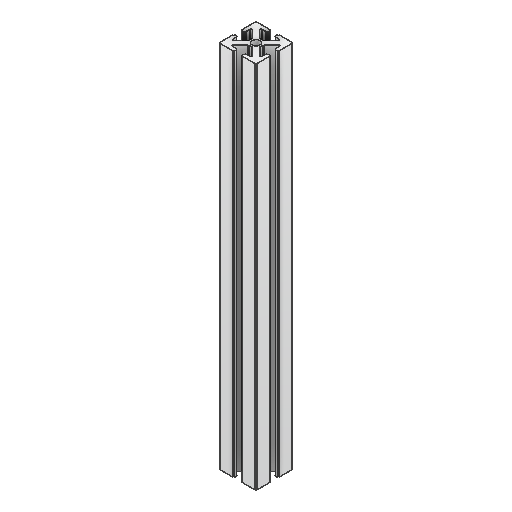
# Autodesk Inventor part: Strut_short
Saved by Autodesk Inventor 2025.2 (Build 292293000, 293)
## iProperties
Created: 2024-10-24
Part Number: Strut_short
Material: Generic
Document SubType Name: Modeling
Designer: rolan
Density: 1 g/cm^3
Appearance: Default
Author: rolan
Autodesk Inventor part; units mm, degrees
ref_plane "YZ Plane" through (0, 0, 0) normal (1, 0, 0) x (0, 1, 0)
ref_plane "XZ Plane" through (0, 0, 0) normal (0, 1, 0) x (-1, 0, 0)
ref_plane "XY Plane" through (0, 0, 0) normal (0, 0, 1) x (1, 0, 0)
sketch "Sketch1" plane through (0, 0, 0) normal (0, 1, 0) x (-1, 0, 0)
  line L0 (2.5, 10) -> (9.5, 10) construction
  line L1 (10, -2.5) -> (10, -9.5) construction
  line L2 (-2.5, -10) -> (-9.5, -10) construction
  line L3 (-10, 2.5) -> (-10, 10) construction
  line L4 (-10, 10) -> (10, -10) construction
  line L5 (10, 10) -> (-10, -10) construction
  circle A0 centre (0, 0) radius 2.15
  line L6 (10, 9.5) -> (10, 2.5)
  line L7 (9.5, 2) -> (8.5, 2)
  line L8 (8, 2.5) -> (8, 4.7929)
  line L9 (-0.7929, 3) -> (0.7929, 3)
  line L10 (3, 0.7929) -> (3, -0.7929)
  line L11 (0.7929, -3) -> (-0.7929, -3)
  line L12 (-3, -0.7929) -> (-3, 0.7929)
  line L13 (-3, 3) -> (3, -3) construction
  line L14 (3, 3) -> (-3, -3) construction
  line L15 (10, -10) -> (10, -2)
  line L16 (9.5, -2) -> (8.5, -2)
  line L17 (8, -2.5) -> (8, -4.7929)
  line L18 (7.1464, -5.1464) -> (3.1464, -1.1464)
  line L19 (7.1464, 5.1464) -> (3.1464, 1.1464)
  line L20 (8, 6) -> (13.6569, 6) construction
  line L21 (10, 10) -> (2, 10)
  line L22 (2, 9.5) -> (2, 8.5)
  line L23 (2.5, 8) -> (4.7929, 8)
  line L24 (5.1464, 7.1464) -> (1.1464, 3.1464)
  line L25 (-9.5, 10) -> (-2.5, 10)
  line L26 (-2, 9.5) -> (-2, 8.5)
  line L27 (-2.5, 8) -> (-4.7929, 8)
  line L28 (-5.1464, 7.1464) -> (-1.1464, 3.1464)
  line L29 (-10, 9.5) -> (-10, 2)
  line L30 (-9.5, 2) -> (-8.5, 2)
  line L31 (-8, 2.5) -> (-8, 4.7929)
  line L32 (-7.1464, 5.1464) -> (-3.1464, 1.1464)
  line L33 (-10, -9.5) -> (-10, -2.5)
  line L34 (-9.5, -2) -> (-8.5, -2)
  line L35 (-8, -2.5) -> (-8, -4.7929)
  line L36 (-7.1464, -5.1464) -> (-3.1464, -1.1464)
  line L37 (-8, -6) -> (-2.3431, -6) construction
  line L38 (-10, -10) -> (-2, -10)
  line L39 (-2, -9.5) -> (-2, -8.5)
  line L40 (-2.5, -8) -> (-4.7929, -8)
  line L41 (-5.1464, -7.1464) -> (-1.1464, -3.1464)
  line L42 (9.5, -10) -> (2.5, -10)
  line L43 (2, -9.5) -> (2, -8.5)
  line L44 (2.5, -8) -> (4.7929, -8)
  line L45 (5.1464, -7.1464) -> (1.1464, -3.1464)
  arc A1 (8, 2.5) -> (8.5, 2) centre (8.5, 2.5) ccw
  arc A2 (9.5, 2) -> (10, 2.5) centre (9.5, 2.5) ccw
  arc A3 (10, -2.5) -> (9.5, -2) centre (9.5, -2.5) ccw
  arc A4 (8.5, -2) -> (8, -2.5) centre (8.5, -2.5) ccw
  arc A5 (7.1464, -5.1464) -> (8, -4.7929) centre (7.5, -4.7929) ccw
  arc A6 (3, -0.7929) -> (3.1464, -1.1464) centre (3.5, -0.7929) ccw
  arc A7 (3.1464, 1.1464) -> (3, 0.7929) centre (3.5, 0.7929) ccw
  arc A8 (8, 4.7929) -> (7.1464, 5.1464) centre (7.5, 4.7929) ccw
  arc A9 (5.1464, 7.1464) -> (4.7929, 8) centre (4.7929, 7.5) ccw
  arc A10 (0.7929, 3) -> (1.1464, 3.1464) centre (0.7929, 3.5) ccw
  arc A11 (-1.1464, 3.1464) -> (-0.7929, 3) centre (-0.7929, 3.5) ccw
  arc A12 (-3, 0.7929) -> (-3.1464, 1.1464) centre (-3.5, 0.7929) ccw
  arc A13 (-3.1464, -1.1464) -> (-3, -0.7929) centre (-3.5, -0.7929) ccw
  arc A14 (-0.7929, -3) -> (-1.1464, -3.1464) centre (-0.7929, -3.5) ccw
  arc A15 (1.1464, -3.1464) -> (0.7929, -3) centre (0.7929, -3.5) ccw
  arc A16 (-4.7929, 8) -> (-5.1464, 7.1464) centre (-4.7929, 7.5) ccw
  arc A17 (-7.1464, 5.1464) -> (-8, 4.7929) centre (-7.5, 4.7929) ccw
  arc A18 (-8, -4.7929) -> (-7.1464, -5.1464) centre (-7.5, -4.7929) ccw
  arc A19 (-5.1464, -7.1464) -> (-4.7929, -8) centre (-4.7929, -7.5) ccw
  arc A20 (4.7929, -8) -> (5.1464, -7.1464) centre (4.7929, -7.5) ccw
  arc A21 (2, 8.5) -> (2.5, 8) centre (2.5, 8.5) ccw
  arc A22 (2.5, 10) -> (2, 9.5) centre (2.5, 9.5) ccw
  arc A23 (-2, 9.5) -> (-2.5, 10) centre (-2.5, 9.5) ccw
  arc A24 (-2.5, 8) -> (-2, 8.5) centre (-2.5, 8.5) ccw
  arc A25 (-10, 2.5) -> (-9.5, 2) centre (-9.5, 2.5) ccw
  arc A26 (-8.5, 2) -> (-8, 2.5) centre (-8.5, 2.5) ccw
  arc A27 (-8, -2.5) -> (-8.5, -2) centre (-8.5, -2.5) ccw
  arc A28 (-9.5, -2) -> (-10, -2.5) centre (-9.5, -2.5) ccw
  arc A29 (-2.5, -10) -> (-2, -9.5) centre (-2.5, -9.5) ccw
  arc A30 (-2, -8.5) -> (-2.5, -8) centre (-2.5, -8.5) ccw
  arc A31 (2, -9.5) -> (2.5, -10) centre (2.5, -9.5) ccw
  arc A32 (2.5, -8) -> (2, -8.5) centre (2.5, -8.5) ccw
  arc A33 (9.5, -10) -> (10, -9.5) centre (9.5, -9.5) ccw
  arc A34 (10, 9.5) -> (9.5, 10) centre (9.5, 9.5) ccw
  arc A35 (-9.5, 10) -> (-10, 9.5) centre (-9.5, 9.5) ccw
  arc A36 (-10, -9.5) -> (-9.5, -10) centre (-9.5, -9.5) ccw
  point P0 (10, 2)
  point P1 (8, 2)
  point P2 (8, -2)
  point P3 (8, -6)
  point P4 (2, 8)
  point P5 (6, 8)
  point P6 (-2, 10)
  point P7 (-2, 8)
  point P8 (-6, 8)
  point P9 (-8, 2)
  point P10 (-8, 6)
  point P11 (-10, -2)
  point P12 (-8, -2)
  point P13 (-2, -8)
  point P14 (-6, -8)
  point P15 (2, -10)
  point P16 (2, -8)
  point P17 (6, -8)
  point P18 (1, 3)
  point P19 (3, 1)
  point P20 (3, -1)
  point P21 (1, -3)
  point P22 (-1, -3)
  point P23 (-3, -1)
  point P24 (-3, 1)
  point P25 (-1, 3)
  dimension "d0" = 20
  dimension "d1" = 20
  dimension "d2" = 4.3
  dimension "d3" = 8
  dimension "d4" = 2
  dimension "d5" = 4
  dimension "d6" = 6
  dimension "d7" = 6
  dimension "d8" = 8
  dimension "d9" = 2
  dimension "d10" = 4
  dimension "d11" = 45
  dimension "d12" = 135
  dimension "d13" = 8
  dimension "d14" = 2
  dimension "d15" = 4
  dimension "d16" = 45
  dimension "d17" = 8
  dimension "d18" = 2
  dimension "d19" = 4
  dimension "d20" = 45
  dimension "d21" = 8
  dimension "d22" = 2
  dimension "d23" = 4
  dimension "d24" = 45
  dimension "d25" = 8
  dimension "d26" = 2
  dimension "d27" = 4
  dimension "d28" = 45
  dimension "d29" = 8
  dimension "d30" = 2
  dimension "d31" = 4
  dimension "d32" = 45
  dimension "d33" = 8
  dimension "d34" = 2
  dimension "d35" = 4
  dimension "d36" = 45
  dimension "d37" = 2
  dimension "d38" = 2
  dimension "d39" = 2
  dimension "d40" = 2
  dimension "d41" = 0.5
  constraints: 92 end point, 80 point on line, 72 point on circle, 72 tangent, 37 centre point, 35 equal radius, 17 perpendicular, 4 horizontal, 4 midpoint, 4 parallel, 2 equal length, 1 coincident, 1 vertical
  measures "d0" distance of L4.end L5.end
  measures "d1" distance of L5.start L4.end
  measures "d2" diameter of A0
  measures "d3" distance of L5.start point (10, 2)
  measures "d4" distance of point (10, 2) point (8, 2)
  measures "d5" distance of point (8, 2) L20.start
  measures "d6" distance of L13.end L14.end
  measures "d7" distance of L14.start L13.end
  measures "d8" distance of L4.end L15.end
  measures "d9" distance of L15.end point (8, -2)
  measures "d10" distance of point (8, -2) point (8, -6)
  measures "d11" angle of L17 L18
  measures "d12" angle of L19 L20
  measures "d13" distance of L5.start L21.end
  measures "d14" distance of L21.end point (2, 8)
  measures "d15" distance of point (2, 8) point (6, 8)
  measures "d16" angle of L23 L24
  measures "d17" distance of L3.end point (-2, 10)
  measures "d18" distance of point (-2, 10) point (-2, 8)
  measures "d19" distance of point (-2, 8) point (-6, 8)
  measures "d20" angle of L28 L27
  measures "d21" distance of L3.end L29.end
  measures "d22" distance of L29.end point (-8, 2)
  measures "d23" distance of point (-8, 2) point (-8, 6)
  measures "d24" angle of L31 L32
  measures "d25" distance of L5.end point (-10, -2)
  measures "d26" distance of point (-10, -2) point (-8, -2)
  measures "d27" distance of point (-8, -2) L37.start
  measures "d28" angle of L37 L36
  measures "d29" distance of L5.end L38.end
  measures "d30" distance of L38.end point (-2, -8)
  measures "d31" distance of point (-2, -8) point (-6, -8)
  measures "d32" angle of L40 L41
  measures "d33" distance of L4.end point (2, -10)
  measures "d34" distance of point (2, -10) point (2, -8)
  measures "d35" distance of point (2, -8) point (6, -8)
  measures "d36" angle of L45 L44
  measures "d37" distance of point (-1, 3) point (1, 3)
  measures "d38" distance of point (3, 1) point (3, -1)
  measures "d39" distance of point (1, -3) point (-1, -3)
  measures "d40" distance of point (-3, -1) point (-3, 1)
  measures "d41" radius of A1
extrude "Extrusion1" add sketch "Sketch1" along normal blind 200
body "Solid1"
